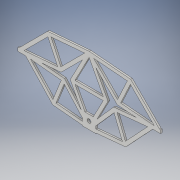
# Autodesk Inventor part: Eye Truss 2
Saved by Autodesk Inventor 2018 (Build 220112000, 112)
## iProperties
Created: 2019-01-14
Part Number: Eye Truss 2
Material: Generic
Document SubType Name: Modeling
Designer: 871357
Density: 1 g/cm^3
Appearance: Default
Author: 871357
Autodesk Inventor part; units mm, degrees
ref_plane "YZ Plane" through (0, 0, 0) normal (1, 0, 0) x (0, 1, 0)
ref_plane "XZ Plane" through (0, 0, 0) normal (0, 1, 0) x (-1, 0, 0)
ref_plane "XY Plane" through (0, 0, 0) normal (0, 0, 1) x (1, 0, 0)
sketch "Sketch1" plane through (0, 0, 0) normal (0, 0, 1) x (1, 0, 0)
  line L0 (0, 0) -> (266.7, 0) construction
  line L1 (266.7, 0) -> (266.7, 127) construction
  line L2 (266.7, 127) -> (0, 127) construction
  line L3 (0, 127) -> (0, 0) construction
  line L4 (3.175, 63.5) -> (57.1495, 117.4745) construction
  line L5 (3.175, 63.5) -> (61.6477, 63.5) construction
  line L6 (133.35, 123.825) -> (209.5505, 117.4745) construction
  line L7 (133.35, 123.825) -> (154.8013, 123.825) construction
  line L8 (133.35, 123.825) -> (57.1495, 117.4745) construction
  line L9 (133.35, 123.825) -> (241.0197, 123.825) construction
  line L10 (133.35, 123.825) -> (79.3755, 69.8505) construction
  line L11 (3.175, 63.5) -> (79.3755, 69.8505) construction
  line L12 (3.175, 63.5) -> (58.3803, 63.5) construction
  line L13 (57.1495, 117.4745) -> (79.3755, 69.8505) construction
  line L14 (263.525, 63.5) -> (334.0804, 63.5) construction
  line L15 (263.525, 63.5) -> (356.1825, 63.5) construction
  line L16 (263.525, 63.5) -> (209.5505, 117.4745) construction
  line L17 (133.35, 123.825) -> (187.3245, 69.8505) construction
  line L18 (263.525, 63.5) -> (187.3245, 69.8505) construction
  line L19 (263.525, 63.5) -> (382.9611, 63.5) construction
  line L20 (187.3245, 69.8505) -> (209.5505, 117.4745) construction
  line L21 (101.6, 63.5) -> (165.1, 63.5) construction
  line L22 (133.35, 123.825) -> (101.6, 63.5) construction
  line L23 (165.1, 63.5) -> (133.35, 123.825) construction
  line L24 (101.6, 63.5) -> (133.35, 3.175) construction
  line L25 (133.35, 3.175) -> (165.1, 63.5) construction
  line L26 (133.35, 3.175) -> (85.725, 56.7523) construction
  line L27 (133.35, 3.175) -> (205.0345, 3.175) construction
  line L28 (133.35, 3.175) -> (233.6369, 3.175) construction
  line L29 (133.35, 3.175) -> (66.675, 9.2359) construction
  line L30 (133.35, 3.175) -> (200.2999, 3.175) construction
  line L31 (66.675, 9.2359) -> (85.725, 56.7523) construction
  line L32 (3.175, 63.5) -> (15.875, 63.5) construction
  line L33 (15.875, 63.5) -> (66.675, 9.2359) construction
  line L34 (85.725, 56.7523) -> (15.875, 63.5) construction
  line L35 (133.35, 3.175) -> (133.35, 50.0944) construction
  line L36 (133.35, 3.175) -> (180.975, 56.7523) construction
  line L37 (133.35, 3.175) -> (200.025, 9.2359) construction
  line L38 (200.025, 9.2359) -> (180.975, 56.7523) construction
  line L39 (263.525, 63.5) -> (250.825, 63.5) construction
  line L40 (250.825, 63.5) -> (200.025, 9.2359) construction
  line L41 (180.975, 56.7523) -> (250.825, 63.5) construction
  line L42 (120.65, 0) -> (146.05, 0)
  circle A0 centre (133.35, 14.1798) radius 3.5449
  line L43 (0, 60.325) -> (14.4981, 60.325)
  line L44 (11.549, 67.3839) -> (56.1894, 112.0242)
  line L45 (56.1894, 112.0242) -> (74.5717, 72.6362)
  line L46 (74.5717, 72.6362) -> (11.549, 67.3839)
  line L47 (61.9533, 114.6888) -> (124.976, 119.9411)
  line L48 (124.976, 119.9411) -> (80.3356, 75.3008)
  line L49 (80.3356, 75.3008) -> (61.9533, 114.6888)
  line L50 (133.35, 127) -> (55.7148, 120.5299)
  line L51 (0, 66.675) -> (1.8599, 66.675)
  line L52 (1.8599, 66.675) -> (55.7148, 120.5299)
  line L53 (120.7865, 106.7714) -> (80.7982, 66.7831)
  line L54 (80.7982, 66.7831) -> (45.4253, 63.8351)
  line L55 (87.2703, 59.7928) -> (45.4253, 63.8351)
  line L56 (87.2703, 59.7928) -> (118.3878, 24.7862)
  line L57 (81.2007, 53.9995) -> (23.9397, 59.5311)
  line L58 (23.9397, 59.5311) -> (65.5841, 15.0469)
  line L59 (81.2007, 53.9995) -> (65.5841, 15.0469)
  line L60 (14.4981, 60.325) -> (65.1701, 6.1977)
  line L61 (0, 66.675) -> (0, 60.325)
  line L62 (120.65, 1.1544) -> (65.1701, 6.1977)
  line L63 (71.2137, 12.0245) -> (86.762, 50.8067)
  line L64 (86.762, 50.8067) -> (120.65, 12.6833)
  line L65 (71.2137, 12.0245) -> (120.65, 7.5306)
  line L66 (120.65, 0) -> (120.65, 1.1544)
  line L67 (120.65, 12.6833) -> (120.65, 7.5306)
  line L68 (98.0121, 63.5) -> (118.3878, 24.7862)
  line L69 (98.0121, 63.5) -> (120.7865, 106.7714)
  line L70 (106.859, 60.325) -> (125.5486, 24.8146)
  line L71 (106.859, 66.675) -> (133.35, 117.008)
  line L72 (125.5486, 24.8146) -> (141.1514, 24.8146)
  line L73 (106.859, 60.325) -> (133.35, 60.325)
  line L74 (106.859, 66.675) -> (133.35, 66.675)
  line L75 (266.7, 60.325) -> (252.2019, 60.325)
  line L76 (255.151, 67.3839) -> (210.5106, 112.0242)
  line L77 (210.5106, 112.0242) -> (192.1283, 72.6362)
  line L78 (192.1283, 72.6362) -> (255.151, 67.3839)
  line L79 (204.7467, 114.6888) -> (141.724, 119.9411)
  line L80 (141.724, 119.9411) -> (186.3644, 75.3008)
  line L81 (186.3644, 75.3008) -> (204.7467, 114.6888)
  line L82 (133.35, 127) -> (210.9852, 120.5299)
  line L83 (266.7, 66.675) -> (264.8401, 66.675)
  line L84 (264.8401, 66.675) -> (210.9852, 120.5299)
  line L85 (145.9135, 106.7714) -> (185.9018, 66.7831)
  line L86 (185.9018, 66.7831) -> (221.2747, 63.8351)
  line L87 (179.4297, 59.7928) -> (221.2747, 63.8351)
  line L88 (179.4297, 59.7928) -> (148.3122, 24.7862)
  line L89 (185.4993, 53.9995) -> (242.7603, 59.5311)
  line L90 (242.7603, 59.5311) -> (201.1159, 15.0469)
  line L91 (185.4993, 53.9995) -> (201.1159, 15.0469)
  line L92 (252.2019, 60.325) -> (201.5299, 6.1977)
  line L93 (146.05, 1.1544) -> (201.5299, 6.1977)
  line L94 (195.4863, 12.0245) -> (179.938, 50.8067)
  line L95 (179.938, 50.8067) -> (146.05, 12.6833)
  line L96 (195.4863, 12.0245) -> (146.05, 7.5306)
  line L97 (168.6879, 63.5) -> (148.3122, 24.7862)
  line L98 (168.6879, 63.5) -> (145.9135, 106.7714)
  line L99 (159.841, 60.325) -> (141.1514, 24.8146)
  line L100 (159.841, 66.675) -> (133.35, 117.008)
  line L101 (159.841, 60.325) -> (133.35, 60.325)
  line L102 (159.841, 66.675) -> (133.35, 66.675)
  line L103 (266.7, 66.675) -> (266.7, 60.325)
  line L104 (146.05, 12.6833) -> (146.05, 7.5306)
  line L105 (146.05, 1.1544) -> (146.05, 0)
  dimension "d1" = 266.7
  dimension "d2" = 127
  dimension "d4" = 45
  dimension "d6" = 4.764
  dimension "d7" = 175.236
  dimension "d9" = 4.764
  dimension "d10" = 63.5
  dimension "d11" = 133.35
  dimension "d12" = 3.175
  dimension "d13" = 135
  dimension "d14" = 3.175
  dimension "d17" = 3.175
  dimension "d18" = 63.5
  dimension "d19" = 175.236
  dimension "d20" = 45
  dimension "d21" = 45
  dimension "d22" = 31.75
  dimension "d23" = 31.75
  dimension "d24" = 60.325
  dimension "d25" = 133.35
  dimension "d26" = 3.175
  dimension "d27" = 131.634
  dimension "d29" = 174.806
  dimension "d30" = 66.675
  dimension "d31" = 47.625
  dimension "d32" = 12.7
  dimension "d33" = 120.65
  dimension "d34" = 25.4
  dimension "d37" = 14.1798
  dimension "d38" = 7.0899
  dimension "d46" = 3.175
  dimension "d47" = 3.175
  dimension "d48" = 3.175
  dimension "d49" = 3.175
  dimension "d50" = 3.175
  dimension "d53" = 6.35
  dimension "d55" = 6.35
  dimension "d56" = 6.35
  dimension "d57" = 3.175
  dimension "d58" = 6.35
  dimension "d59" = 6.35
  dimension "d60" = 3.175
  dimension "d61" = 3.175
  dimension "d62" = 6.35
  dimension "d63" = 3.175
  dimension "d67" = 6.35
  dimension "d68" = 3.175
  dimension "d69" = 6.35
  dimension "d70" = 6.35
  dimension "d71" = 6.35
  dimension "d72" = 3.175
  dimension "d73" = 3.175
  dimension "d74" = 6.35
  dimension "d75" = 6.35
  dimension "d76" = 3.175
  dimension "d77" = 26.4911
  dimension "d78" = 6.35
  constraints: 212 end point, 31 symmetric about line, 26 parallel, 16 horizontal, 6 point on line, 3 perpendicular, 2 collinear, 2 equal length, 2 vertical, 1 centre point, 1 midpoint
  measures "d1" distance of L2.end L1.end
  measures "d2" distance of L1.end L0.end
  measures "d4" angle of L5 L4
  measures "d6" angle of L6 L7
  measures "d7" angle of L8 L9
  measures "d9" angle of L12 L11
  measures "d10" vertical distance of L2.end L4.start
  measures "d11" horizontal distance of L6.start L2.end
  measures "d12" distance from line of L2 L6.start
  measures "d13" angle of L9 L10
  measures "d14" horizontal distance of L4.start L2.end
  measures "d17" distance from line of L1 L14.start
  measures "d18" distance from line of L2 L14.start
  measures "d19" angle of L19 L18
  measures "d20" angle of L9 L17
  measures "d21" angle of L9 L16
  measures "d22" horizontal distance of L6.start L21.end
  measures "d23" horizontal distance of L6.start L21.start
  measures "d24" distance from line of L21 L6.start
  measures "d25" horizontal distance of L0.start L24.end
  measures "d26" distance from line of L0 L24.end
  measures "d27" angle of L27 L26
  measures "d29" angle of L30 L29
  measures "d30" horizontal distance of L24.end L29.end
  measures "d31" horizontal distance of L24.end L26.end
  measures "d32" distance of L4.start L32.end
  measures "d33" distance from line of L1 L42.end
  measures "d34" distance of L42.start L42.end
  measures "d37" distance from line of L0 A0.centre
  measures "d38" diameter of A0
  measures "d46" distance between parallel lines of L13 L45
  measures "d47" distance between parallel lines of L11 L46
  measures "d48" distance between parallel lines of L8 L47
  measures "d49" distance between parallel lines of L10 L48
  measures "d50" distance between parallel lines of L13 L49
  measures "d53" diameter of L43 L5
  measures "d55" distance between parallel lines of L43 L51
  measures "d56" distance between parallel lines of L44 L52
  measures "d57" distance between parallel lines of L4 L52
  measures "d58" distance between parallel lines of L54 L46
  measures "d59" distance between parallel lines of L48 L53
  measures "d60" distance between parallel lines of L55 L34
  measures "d61" distance between parallel lines of L26 L56
  measures "d62" distance between parallel lines of L55 L57
  measures "d63" distance between parallel lines of L31 L59
  measures "d67" distance between parallel lines of L58 L60
  measures "d68" distance between parallel lines of L58 L33
  measures "d69" distance between parallel lines of L59 L63
  measures "d70" distance between parallel lines of L56 L64
  measures "d71" distance between parallel lines of L62 L65
  measures "d72" distance between parallel lines of L24 L68
  measures "d73" distance between parallel lines of L22 L69
  measures "d74" distance between parallel lines of L68 L70
  measures "d75" distance between parallel lines of L69 L71
  measures "d76" distance between parallel lines of L21 L73
  measures "d77" distance of L70.start L73.end
  measures "d78" distance between parallel lines of L73 L74
extrude "Extrusion1" add sketch "Sketch1" along normal blind 3.175
body "Solid1"
